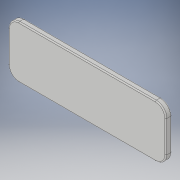
# Autodesk Inventor part: Tabs .5 inch
Saved by Autodesk Inventor 2017.3 (Build 213256000, 256)
## iProperties
Created: 2019-02-15
Part Number: Tabs .5 inch
Material: Generic
Document SubType Name: Modeling
Designer: LSabe
Density: 1 g/cm^3
Appearance: Default
Author: LSabe
Autodesk Inventor part; units mm, degrees
ref_plane "YZ Plane" through (0, 0, 0) normal (1, 0, 0) x (0, 1, 0)
ref_plane "XZ Plane" through (0, 0, 0) normal (0, 1, 0) x (-1, 0, 0)
ref_plane "XY Plane" through (0, 0, 0) normal (0, 0, 1) x (1, 0, 0)
sketch "Sketch1" plane through (0, 0, 0) normal (0, 0, 1) x (1, 0, 0)
  line L0 (0, 0) -> (38.1, 0)
  line L1 (38.1, 0) -> (38.1, 12.7)
  line L2 (38.1, 12.7) -> (0, 12.7)
  line L3 (0, 12.7) -> (0, 0)
  constraints: 8 end point, 2 parallel, 1 horizontal, 1 perpendicular
extrude "Extrusion1" add sketch "Sketch1" along normal blind 1.397
fillet "Fillet1" radius 2.54 4 edges at (0, 12.7, 0.6985) (38.1, 12.7, 0.6985) (38.1, 0, 0.6985) (0, 0, 0.6985)
fillet "Fillet2" radius 0.254 16 edges at (0.7439, 11.9561, 0) (0, 6.35, 0) (0.7439, 0.7439, 0) (19.05, 0, 0) (37.3561, 0.7439, 0) (38.1, 6.35, 0) (37.3561, 11.9561, 0) (19.05, 12.7, 0) (0.7439, 11.9561, 1.397) (0, 6.35, 1.397) (0.7439, 0.7439, 1.397) (19.05, 0, 1.397) (37.3561, 0.7439, 1.397) (38.1, 6.35, 1.397) (37.3561, 11.9561, 1.397) (19.05, 12.7, 1.397)
body "Solid1"
